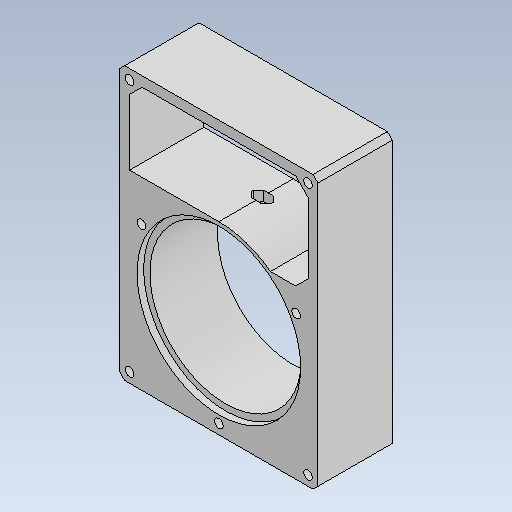
# Autodesk Inventor part: housing_3dp
Saved by Autodesk Inventor 2026.1 (Build 301233020, 233B)
## iProperties
Created: 2026-08-16
Part Number: housing_3dp
Material: 一般
Document SubType Name: Modeling
Designer: ug_nd
Density: 1 g/cm^3
Appearance: 既定
Author: ug_nd
Autodesk Inventor part; units mm, degrees
ref_plane "YZ Plane" through (0, 0, 0) normal (1, 0, 0) x (0, 1, 0)
ref_plane "XZ Plane" through (0, 0, 0) normal (0, 1, 0) x (-1, 0, 0)
sketch "スケッチ1" plane through (0, 0, 0) normal (0, 0, 1) x (1, 0, 0)
  line L0 (38, -55) -> (-38, -55)
  line L1 (-40, -53) -> (-40, 53)
  line L2 (-38, 55) -> (38, 55)
  line L3 (40, 53) -> (40, -53)
  line L4 (40, -55) -> (-40, 55) construction
  line L5 (-40, -55) -> (40, 55) construction
  line L6 (-38, 55) -> (-40, 53)
  line L7 (38, 55) -> (40, 53)
  line L8 (40, -53) -> (38, -55)
  line L9 (-38, -55) -> (-40, -53)
  circle A0 centre (-36, 51) radius 1.75
  line L10 (-56, 0) -> (56, 0) construction
  line L11 (0, -77) -> (0, 77) construction
  circle A1 centre (36, 51) radius 1.75
  circle A2 centre (-36, -51) radius 1.75
  circle A3 centre (36, -51) radius 1.75
  line L12 (31, -51) -> (-31, -51)
  line L13 (-36, -46) -> (-36, 46)
  line L14 (-31, 51) -> (31, 51)
  line L15 (36, 46) -> (36, -46)
  line L16 (36, -51) -> (-36, 51) construction
  line L17 (-36, -51) -> (36, 51) construction
  line L18 (-31, 51) -> (-36, 46)
  line L19 (36, 46) -> (31, 51)
  line L20 (-31, -51) -> (-36, -46)
  line L21 (31, -51) -> (36, -46)
  point P0 (0, 0)
  dimension "d1" = 80
  dimension "d2" = 110
  dimension "d3" = 2
  dimension "d4" = 2
  dimension "d5" = 2
  dimension "d6" = 2
  dimension "d7" = 2
  dimension "d8" = 2
  dimension "d9" = 2
  dimension "d10" = 2
  dimension "d11" = 3.5
  dimension "d12" = 4
  dimension "d13" = 4
  dimension "d14" = 4
  dimension "d15" = 4
  dimension "d16" = 5
  dimension "d17" = 5
  dimension "d18" = 5
  dimension "d19" = 5
  dimension "d20" = 5
  dimension "d21" = 5
  dimension "d22" = 5
  dimension "d23" = 5
  constraints: 40 end point, 16 point on line, 4 centre point, 4 midpoint, 4 parallel, 3 symmetric about line, 2 horizontal, 2 perpendicular, 3 other
  measures "d1" distance between parallel lines of L3 L1
  measures "d2" distance between parallel lines of L0 L2
  measures "d3" distance of L2.start L4.end
  measures "d4" distance of L1.end L4.end
  measures "d5" distance of L2.end L5.end
  measures "d6" distance of L3.start L5.end
  measures "d7" distance of L3.end L4.start
  measures "d8" distance of L0.start L4.start
  measures "d9" distance of L0.end L5.start
  measures "d10" distance of L1.start L5.start
  measures "d11" diameter of A0
  measures "d12" distance from line of L2 A0.centre
  measures "d13" distance from line of L1 A0.centre
  measures "d14" distance between parallel lines of L2 L14
  measures "d15" distance between parallel lines of L1 L13
  measures "d16" distance of L14.start L16.end
  measures "d17" distance of L13.end L16.end
  measures "d18" distance of L15.start L17.end
  measures "d19" distance of L14.end L17.end
  measures "d20" distance of L12.end L17.start
  measures "d21" distance of L13.start L17.start
  measures "d22" distance of L12.start L16.start
  measures "d23" distance of L15.end L16.start
extrude "押し出し1" add sketch "スケッチ1" against normal blind 30
ref_plane "作業平面1" through (0, 0, -2.7) normal (0, 0, 1) x (1, 0, 0)
sketch "スケッチ2" plane through (0, 0, -2.7) normal (0, 0, 1) x (1, 0, 0)
  line L0 (-56, 0) -> (56, 0) construction
  line L1 (0, -77) -> (0, 77) construction
  circle A0 centre (0, -15) radius 36 construction
  line L2 (31, -51) -> (-31, -51) projected
  circle A1 centre (0, -15) radius 30.5
  line L3 (-36, 20) -> (4, 20) construction
  line L4 (4, 20) -> (4, 36) construction
  line L5 (4, 36) -> (-36, 36) construction
  line L6 (-36, 36) -> (-36, 20) construction
  line L7 (-36, 20) -> (4, 36) construction
  line L8 (4, 20) -> (-36, 36) construction
  line L9 (-36, 46) -> (-31, 51) construction
  line L10 (-31, 51) -> (31, 51) construction
  line L11 (31, 51) -> (36, 46) construction
  line L12 (36, 46) -> (36, -46) construction
  line L13 (36, -46) -> (31, -51) projected
  line L14 (-31, -51) -> (-36, -46) projected
  line L15 (-36, -46) -> (-36, 46) construction
  circle A2 centre (25, 25) radius 12.5 construction
  circle A3 centre (0, -15) radius 34.5 construction
  line L16 (0, 19.5) -> (-36, 19.5)
  arc A4 (20.8327, 12.5) -> (0, 19.5) centre (0, -15) ccw
  line L17 (20.8327, 12.5) -> (31, 12.5)
  line L18 (-36, 19.5) -> (-36, -46)
  line L19 (36, 17.5) -> (36, -46)
  line L20 (31, 12.5) -> (36, 17.5)
  point P0 (0, 0)
  point P1 (-16, 28)
  point P2 (36, 12.5)
  dimension "d27" = 72
  dimension "d28" = 61
  dimension "d29" = 35
  dimension "d30" = 4
  dimension "d31" = 40
  dimension "d32" = 16
  dimension "d33" = 4
  dimension "d34" = 25
  dimension "d35" = 40
  dimension "d36" = 25
  dimension "d39" = 5
  dimension "d40" = 5
  constraints: 22 end point, 6 point on line, 5 centre point, 4 point on circle, 3 horizontal, 2 coincident, 2 midpoint, 2 parallel, 2 tangent, 1 concentric, 1 perpendicular
  measures "d27" diameter of A0
  measures "d28" diameter of A1
  measures "d29" distance from line of A0.centre L3
  measures "d30" distance between parallel lines of L1 L4
  measures "d31" distance of L4.end L5.end
  measures "d32" distance of L3.end L4.end
  measures "d33" radial gap between concentric circles of A3 A1
  measures "d34" diameter of A2
  measures "d35" vertical distance of A0.centre A2.centre
  measures "d36" distance from line of L1 A2.centre
  measures "d39" distance of L17.end point (36, 12.5)
  measures "d40" distance of L19.start point (36, 12.5)
extrude "押し出し2" add sketch "スケッチ2" against normal up to surface (27.3 mm away)
sketch "スケッチ3" plane through (0, 0, -2.7) normal (0, 0, 1) x (1, 0, 0)
  line L0 (0, 19.5) -> (-36, 19.5) projected
  line L1 (-36, -46) -> (-36, 19.5) projected
  line L2 (-31, -51) -> (-36, -46) projected
  line L3 (31, -51) -> (-31, -51) projected
  line L4 (36, -46) -> (31, -51) projected
  line L5 (36, 17.5) -> (36, -46) projected
  line L6 (36, 17.5) -> (31, 12.5) projected
  line L7 (31, 12.5) -> (20.8327, 12.5) projected
  arc A0 (20.8327, 12.5) -> (0, 19.5) centre (0, -15) ccw projected
  circle A1 centre (0, -15) radius 30.5 construction
  circle A2 centre (0, -15) radius 33
  point P0 (0, 0)
  dimension "d41" = 66
  constraints: 1 centre point, 1 coincident
  measures "d41" diameter of A2
extrude "押し出し3" add sketch "スケッチ3" along normal up to surface (2.7 mm away)
sketch "スケッチ4" plane through (0, 0, 0) normal (0, 0, 1) x (1, 0, 0)
  circle A0 centre (0, -15) radius 30.5 construction
  circle A1 centre (0, -15) radius 36 construction
  line L0 (0, -77) -> (0, 77) construction
  circle A2 centre (0, -51) radius 1.75
  circle A3 centre (31.1769, 3) radius 1.75
  circle A4 centre (-31.1769, 3) radius 1.75
  point P0 (0, 0)
  dimension "d44" = 72
  dimension "d45" = 3.5
  dimension "d48" = 360
  constraints: 3 centre point, 1 coincident, 1 point on line, 1 vertical alignment, 9 other
  measures "d45" diameter of A2
extrude "押し出し4" cut sketch "スケッチ4" against normal through all
sketch "スケッチ5" plane through (0, 0, -30) normal (0, 0, -1) x (-1, 0, 0)
  circle A0 centre (-31.1769, 3) radius 1.75 construction
  circle A1 centre (31.1769, 3) radius 1.75 construction
  circle A2 centre (0, -51) radius 1.75 construction
  line L0 (-29.5603, 5.8) -> (-27.9438, 3)
  line L1 (-27.9438, 3) -> (-29.5603, 0.2)
  line L2 (-29.5603, 0.2) -> (-32.7935, 0.2)
  line L3 (-32.7935, 0.2) -> (-34.4101, 3)
  line L4 (-34.4101, 3) -> (-32.7935, 5.8)
  line L5 (-32.7935, 5.8) -> (-29.5603, 5.8)
  line L6 (32.7935, 5.8) -> (34.4101, 3)
  line L7 (34.4101, 3) -> (32.7935, 0.2)
  line L8 (32.7935, 0.2) -> (29.5603, 0.2)
  line L9 (29.5603, 0.2) -> (27.9438, 3)
  line L10 (27.9438, 3) -> (29.5603, 5.8)
  line L11 (29.5603, 5.8) -> (32.7935, 5.8)
  line L12 (1.6166, -48.2) -> (3.2332, -51)
  line L13 (3.2332, -51) -> (1.6166, -53.8)
  line L14 (1.6166, -53.8) -> (-1.6166, -53.8)
  line L15 (-1.6166, -53.8) -> (-3.2332, -51)
  line L16 (-3.2332, -51) -> (-1.6166, -48.2)
  line L17 (-1.6166, -48.2) -> (1.6166, -48.2)
  point P0 (0, 0)
  dimension "d52" = 5.6
  constraints: 36 end point, 3 coincident, 3 horizontal, 2 equal length, 39 other
  measures "d52" distance between parallel lines of L13 L16
extrude "押し出し5" cut sketch "スケッチ5" against normal blind 5
sketch "スケッチ6" plane through (0, 0, 0) normal (0, 1, 0) x (-1, 0, 0)
  line L0 (-4, -20) -> (4, -20)
  line L1 (4, -20) -> (4, -15)
  line L2 (4, -15) -> (-4, -15)
  line L3 (-4, -15) -> (-4, -20)
  line L4 (-4, -20) -> (4, -15) construction
  line L5 (4, -20) -> (-4, -15) construction
  line L6 (0, -62.7735) -> (0, 10.4622) construction
  line L7 (56, 0) -> (-56, 0) construction
  point P0 (0, 0)
  point P1 (0, -17.5)
  dimension "d55" = 5
  dimension "d56" = 8
  dimension "d57" = 17.5
  constraints: 12 end point, 2 midpoint, 2 parallel, 1 horizontal, 1 perpendicular, 1 point on line
  measures "d55" distance of L2.end L0.start
  measures "d56" distance of L0.start L0.end
  measures "d57" distance from line of L7 point (0, -17.5)
extrude "押し出し6" cut sketch "スケッチ6" along normal up to surface (19.5 mm away)
chamfer "面取り1" distance 2 angle 45 4 edges at (-4, 17.3683, -20) (-4, 17.3683, -15) (4, 17.2519, -15) (4, 17.2519, -20)
equation "\"d4\" = d3"
equation "\"d5\" = d3"
equation "\"d6\" = d5"
equation "\"d7\" = d3"
equation "\"d8\" = d7"
equation "\"d9\" = d3"
equation "\"d10\" = d9"
equation "\"d17\" = d16"
equation "\"d19\" = d18"
equation "\"d20\" = d18"
equation "\"d21\" = d20"
equation "\"d22\" = d18"
equation "\"d23\" = d22"
equation "\"d40\" = d39"
